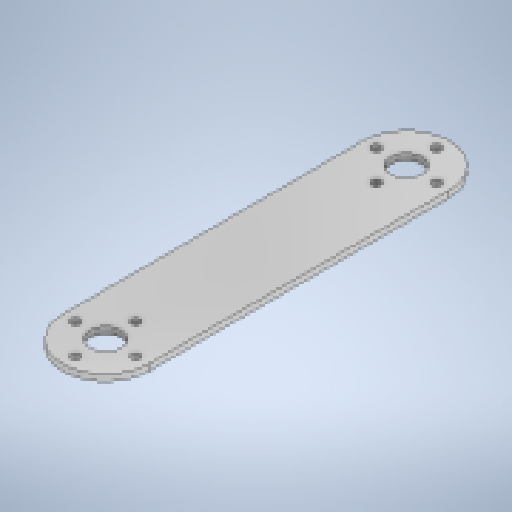
# Autodesk Inventor part: axis_10_11-connector_frame
Saved by Autodesk Inventor 2025.2 (Build 292293000, 293)
## iProperties
Created: 2025-05-04
Part Number: axis_10_11-connector_frame
Material: Aluminum 6061-AHC
Document SubType Name: Sheet Metal
Designer: User
Density: 2.7 g/cm^3
Sheet Metal Rule: Default_mm
Appearance: Aluminum - Dark
Author: User
Autodesk Inventor part; units mm, degrees
ref_plane "YZ Plane" through (0, 0, 0) normal (1, 0, 0) x (0, 1, 0)
ref_plane "XZ Plane" through (0, 0, 0) normal (0, 1, 0) x (-1, 0, 0)
ref_plane "XY Plane" through (0, 0, 0) normal (0, 0, 1) x (1, 0, 0)
sketch "Sketch1" plane through (0, 0, 0) normal (0, 1, 0) x (-1, 0, 0)
  line L0 (10, -45) -> (-10, -45)
  line L1 (-10, -45) -> (-10, 45)
  line L2 (-10, 45) -> (10, 45)
  line L3 (10, 45) -> (10, -45)
  point P0 (0, 0)
  dimension "d0" = 20
  dimension "d1" = 90
  dimension "d2" = 45
  dimension "d3" = 10
  measures "d0" distance of L0.start L0.end
  measures "d1" distance of L0.end L1.end
  measures "d2" distance from line of L0 point (0, 0)
  measures "d3" distance from line of point (0, 0) L1
extrude "Plate1" add sketch "Sketch1" along normal blind 1.5
sketch "Sketch2" plane through (0, 0, 0) normal (0, -1, 0) x (1, 0, 0)
  circle A0 centre (0, 42) radius 0.7835 projected
  circle A1 centre (-7, 35) radius 0.7835 projected
  circle A2 centre (0, 28) radius 0.7835 projected
  circle A3 centre (7, 35) radius 0.7835 projected
  circle A4 centre (0, -28) radius 0.7835 projected
  circle A5 centre (-7, -35) radius 0.7835 projected
  circle A6 centre (0, -42) radius 0.7835 projected
  circle A7 centre (7, -35) radius 0.7835 projected
  point P0 (0, 0)
hole "Hole1" at (0, 0, 42) at (-7, 0, 35) at (0, 0, 28) at (7, 0, 35) at (0, 0, -28) at (-7, 0, -35) at (0, 0, -42) at (7, 0, -35) direction (0, 1, 0) diameter 2.1 depth 1.5
sketch "Sketch3" plane through (0, 1.5, 0) normal (0, 1, 0) x (1, 0, 0)
  arc A0 (10, 35) -> (-10, 35) centre (0, 35) ccw
  arc A1 (-10, -35) -> (10, -35) centre (0, -35) ccw
  line L0 (-10, 35) -> (-10, -35)
  line L1 (10, 35) -> (10, -35)
  line L2 (10, 45) -> (10, -45) projected
  line L3 (-10, 45) -> (10, 45)
  line L4 (10, 45) -> (10, -45)
  line L5 (10, -45) -> (-10, -45)
  line L6 (-10, -45) -> (-10, 45)
  point P0 (0, 0)
  point P1 (0, 45)
  point P2 (10, 35)
  point P3 (-10, -35)
  point P4 (0, -45)
  point P5 (10, -35)
  dimension "d12" = 35
  dimension "d13" = 35
  dimension "d14" = 10
  dimension "d15" = 10
  dimension "d16" = 10
  dimension "d17" = 20
  dimension "d18" = 90
  constraints: 12 end point, 4 point on circle, 4 tangent, 3 parallel, 2 centre point, 1 horizontal, 1 perpendicular
  measures "d12" distance of point (0, 0) A0.centre
  measures "d13" distance of point (0, 0) A1.centre
  measures "d14" radius of A0
  measures "d15" radius of A1
  measures "d16" distance from line of point (0, 0) L1
  measures "d17" distance of L3.start L3.end
  measures "d18" distance of L5.end L3.start
extrude "Extrusion1" cut sketch "Sketch3" against normal blind 10 contours A0 L3 L2 | A0 L6 L3 | L2 L5 A1 | L5 L6 A1
sketch "Sketch4" plane through (0, 0, 0) normal (0, -1, 0) x (1, 0, 0)
  arc A0 (-10, -35) -> (10, -35) centre (0, -35) ccw projected
  arc A1 (10, 35) -> (-10, 35) centre (0, 35) ccw projected
  point P0 (0, 0)
hole "Hole2" at (0, 0, 35) at (0, 0, -35) direction (0, 1, 0) diameter 7.2 depth 1.5
equation "\"d10\" = Thickness"
equation "\"d26\" = Thickness"
equation "\"d4\" = Thickness"
equation "\"BendReliefWidth\" = Thickness"
equation "\"BendReliefDepth\" = 0.5 * Thickness"
equation "\"CornerReliefSize\" = 4 * Thickness"
equation "\"MinimumRemnant\" = 2 * Thickness"
equation "\"TransitionRadius\" = BendRadius"
equation "\"JacobiRadiusSize\" = BendRadius"
equation "\"GapSize\" = Thickness"
equation "\"Thickness\" = 1.5"
equation "\"BendRadius\" = 0.31"
body "Solid1"
